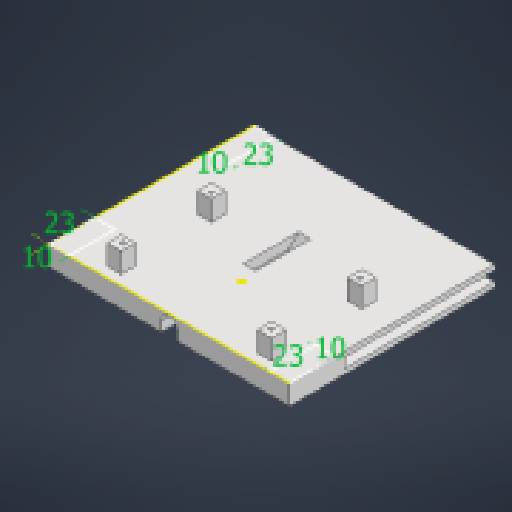
# Autodesk Inventor part: PCB_Housing_01_V3
Saved by Autodesk Inventor 2026.2 (Build 302298000, 298)
## iProperties
Created: 2026-03-09
Part Number: PCB_Housing_01_V3
Material: Generic
Document SubType Name: Modeling
Designer: vckot
Density: 1 g/cm^3
Appearance: Default
Author: vckot
Autodesk Inventor part; units mm, degrees
ref_plane "YZ Plane" through (0, 0, 0) normal (1, 0, 0) x (0, 1, 0)
ref_plane "XZ Plane" through (0, 0, 0) normal (0, 1, 0) x (-1, 0, 0)
ref_plane "XY Plane" through (0, 0, 0) normal (0, 0, 1) x (1, 0, 0)
sketch "Sketch1" plane through (0, 0, 0) normal (0, 1, 0) x (-1, 0, 0)
  line L0 (34, 19) -> (-34, 19)
  line L1 (-34, 19) -> (-34, -19)
  line L2 (-34, -19) -> (34, -19)
  line L3 (34, -19) -> (34, 19)
  line L4 (34, 19) -> (-34, -19) construction
  line L5 (-34, 19) -> (34, -19) construction
  line L6 (41, 26) -> (-41, 26)
  line L7 (-41, 26) -> (-41, -26)
  line L8 (-41, -26) -> (41, -26)
  line L9 (41, -26) -> (41, 26)
  line L10 (41, 26) -> (-41, -26) construction
  line L11 (-41, 26) -> (41, -26) construction
  line L12 (-34, -19) -> (-41, -19)
  line L13 (-34, -19) -> (-34, -26)
  line L14 (-34, 19) -> (-41, 19)
  line L15 (-34, 19) -> (-34, 26)
  line L16 (34, -19) -> (34, -26)
  line L17 (34, -19) -> (41, -19)
  line L18 (34, 19) -> (41, 19)
  line L19 (34, 19) -> (34, 26)
  point P0 (0, 0)
  dimension "d0" = 68
  dimension "d1" = 38
  dimension "d2" = 82
  dimension "d3" = 52
  constraints: 40 end point, 10 point on line, 8 perpendicular, 4 midpoint, 4 parallel, 2 horizontal
  measures "d0" distance of L2.end L1.end
  measures "d1" distance of L1.end L0.end
  measures "d2" distance of L8.end L7.end
  measures "d3" distance of L7.end L6.end
extrude "Extrusion1" add sketch "Sketch1" along normal mid plane 10 contours L19 L6 L9 L18 | L14 L7 L6 L15 | L17 L9 L8 L16 | L13 L8 L7 L12
sketch "Sketch2" plane through (0, -5, 0) normal (0, -1, 0) x (1, 0, 0)
  line L0 (-65, -71.5) -> (55, -71.5)
  line L1 (55, -71.5) -> (55, 31)
  line L2 (55, 31) -> (-65, 31)
  line L3 (-65, 31) -> (-65, -71.5)
  line L4 (-34, 26) -> (-41, 26) projected
  point P0 (0, 0)
  dimension "d6" = 120
  dimension "d7" = 102.5
  dimension "d8" = 5
  dimension "d9" = 55
  constraints: 8 end point, 2 parallel, 1 horizontal, 1 perpendicular
  measures "d6" distance of L1.end L2.end
  measures "d7" distance of L0.end L1.end
  measures "d8" distance between parallel lines of L2 L4
  measures "d9" distance from line of L1 point (0, 0)
extrude "Extrusion2" add sketch "Sketch2" along normal blind 10
sketch "Sketch3" plane through (-65, -5, 31) normal (0, 0, 1) x (1, 0, 0)
  circle A0 centre (60, -5) radius 4
  line L0 (120, -10) -> (0, -10) projected
  line L1 (120, 0) -> (120, -10) projected
  circle A1 centre (60, -5) radius 2.55
  circle A2 centre (60, -5) radius 3
  line L2 (56, -5) -> (56, -10)
  line L3 (64, -5) -> (64, -10)
  line L4 (56, -10) -> (64, -10)
  point P0 (65, 5)
  point P1 (60, -10)
  dimension "d13" = 8
  dimension "d14" = 5
  dimension "d16" = 5.1
  dimension "d17" = 6
  constraints: 6 end point, 3 centre point, 3 perpendicular, 2 coincident, 2 point on circle, 2 point on line, 2 tangent, 1 midpoint, 1 vertical alignment
  measures "d13" diameter of A0
  measures "d14" distance from line of L0 A0.centre
  measures "d16" diameter of A1
  measures "d17" diameter of A2
extrude "Extrusion3" cut sketch "Sketch3" against normal blind 30 contours A0 | L3 L0 L2 A0 | A1 | A2
extrude "Extrusion4" cut sketch "Sketch3" against normal blind 60 contours A1
ref_plane "Work Plane2" through (-65, -5, -4) normal (0, 0, 1) x (1, 0, 0)
sketch "Sketch5" plane through (-65, -5, -4) normal (0, 0, 1) x (1, 0, 0)
  circle A0 centre (60, -5) radius 3 projected
  point P0 (65, 5)
extrude "Extrusion5" cut sketch "Sketch5" against normal up to surface (25 mm away)
sketch "Sketch6" plane through (0, -5, 0) normal (0, 1, 0) x (1, 0, 0)
  line L0 (-2, 4) -> (-2, 29) projected
  line L1 (-2, 29) -> (-8, 29) projected
  line L2 (-8, 4) -> (-8, 29) projected
  line L3 (-2, 9) -> (-8, 9)
  point P0 (0, 0)
  dimension "d25" = 20
  constraints: 2 end point, 2 point on line, 1 perpendicular
  measures "d25" distance between parallel lines of L1 L3
extrude "Extrusion6" cut sketch "Sketch6" against normal blind 5
fillet "Fillet1" [suppressed]
chamfer "Chamfer1" distance 7.5 angle 45 1 edges at (-5, -5, -29)
sketch "Sketch7" plane through (0, 5, 0) normal (0, 1, 0) x (1, 0, 0)
  circle A0 centre (37, 22) radius 1.6 projected
  circle A1 centre (37, -22) radius 1.6 projected
  circle A2 centre (-37, -22) radius 1.6 projected
  point P0 (0, 0)
  point P1 (-37, 22)
  constraints: 1 horizontal alignment, 1 vertical alignment
hole "Hole1" at (37, 5, -22) at (37, 5, 22) at (-37, 5, 22) at (-37, 5, -22) direction (0, -1, 0) diameter 2 depth 8 tip angle 118
sketch "Sketch8" plane through (0, -5, 0) normal (0, 1, 0) x (1, 0, 0)
  line L0 (-65, -31) -> (-55, -31)
  line L1 (-55, -31) -> (-55, -8)
  line L2 (-55, -8) -> (-65, -8)
  line L3 (-65, -8) -> (-65, -31)
  line L4 (-65, -31) -> (-65, 71.5) projected
  line L5 (-65, 71.5) -> (-55, 71.5)
  line L6 (-55, 71.5) -> (-55, 48.5)
  line L7 (-55, 48.5) -> (-65, 48.5)
  line L8 (-65, 48.5) -> (-65, 71.5)
  line L9 (55, -31) -> (-65, -31) projected
  line L10 (55, -31) -> (45, -31)
  line L11 (45, -31) -> (45, -8)
  line L12 (45, -8) -> (55, -8)
  line L13 (55, -8) -> (55, -31)
  point P0 (0, 0)
  dimension "d39" = 10
  dimension "d40" = 23
  dimension "d41" = 10
  dimension "d42" = 23
  dimension "d43" = 10
  dimension "d44" = 23
  constraints: 24 end point, 6 parallel, 3 horizontal, 3 perpendicular
  measures "d39" distance between parallel lines of L3 L1
  measures "d40" distance between parallel lines of L0 L2
  measures "d41" distance of L6.end L7.end
  measures "d42" distance of L5.end L6.end
  measures "d43" distance of L11.end L12.end
  measures "d44" distance of L10.end L11.end
sketch "Sketch9" plane through (55, -5, -71.5) normal (0, 0, -1) x (-1, 0, 0)
  line L0 (120, 0) -> (120, -10) projected
  line L1 (120, -2.5) -> (110, -2.5)
  line L2 (110, -2.5) -> (110, -7.5)
  line L3 (110, -7.5) -> (120, -7.5)
  line L4 (120, -7.5) -> (120, -2.5)
  line L5 (0, 0) -> (0, -10) projected
  line L6 (0, -2.5) -> (10, -2.5)
  line L7 (10, -2.5) -> (10, -7.5)
  line L8 (10, -7.5) -> (0, -7.5)
  line L9 (0, -7.5) -> (0, -2.5)
  point P0 (55, 5)
  point P1 (110, -5)
  point P2 (120, -5)
  point P3 (10, -5)
  point P4 (0, -5)
  point P5 (0, -7.5)
  dimension "d45" = 5
  dimension "d46" = 10
  dimension "d47" = 10
  dimension "d48" = 5
  constraints: 16 end point, 4 midpoint, 4 parallel, 2 horizontal, 2 horizontal alignment, 2 perpendicular, 2 point on line
  measures "d45" distance of L1.end L2.end
  measures "d46" distance of L1.start L1.end
  measures "d47" distance of L7.end L8.end
  measures "d48" distance of L6.end L7.end
extrude "Extrusion7" cut sketch "Sketch9" against normal blind 75
body "Solid1"
